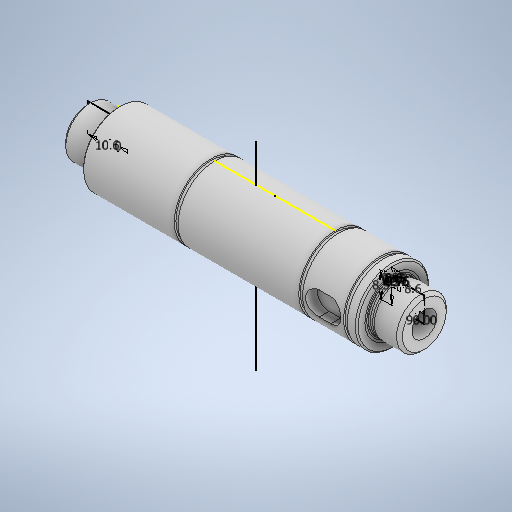
# Autodesk Inventor part: 26-10-204
Saved by Autodesk Inventor 2025.2 (Build 292293000, 293)
## iProperties
Created: 2024-12-02
Part Number: 26-10-204
Material: Generic
Document SubType Name: Modeling
Designer: Zvonko.Gabric
Density: 1 g/cm^3
Appearance: Default
Author: Zvonko.Gabric
Autodesk Inventor part; units mm, degrees
ref_plane "YZ Plane" through (0, 0, 0) normal (1, 0, 0) x (0, 1, 0)
ref_plane "XZ Plane" through (0, 0, 0) normal (0, 1, 0) x (-1, 0, 0)
sketch "Sketch1" plane through (0, 0, 0) normal (0, 1, 0) x (-1, 0, 0)
  line L0 (0, 0) -> (93.8, 0)
  line L1 (0, 9.695) -> (0.1, 8.9835)
  line L2 (0, 12.5) -> (0, 9.695)
  line L3 (3.2, 12.5) -> (0, 12.5)
  line L4 (3.2, 11.95) -> (3.2, 12.5)
  line L5 (4.5, 11.95) -> (3.2, 11.95)
  line L6 (4.5, 12.5) -> (4.5, 11.95)
  line L7 (18.5, 12.5) -> (4.5, 12.5)
  line L8 (18.5, 11.95) -> (18.5, 12.5)
  line L9 (19.8, 11.95) -> (18.5, 11.95)
  line L10 (19.8, 12.5) -> (19.8, 11.95)
  line L11 (61, 12.5) -> (19.8, 12.5)
  line L12 (61, 11.95) -> (61, 12.5)
  line L13 (62.3, 11.95) -> (61, 11.95)
  line L14 (62.3, 12.5) -> (62.3, 11.95)
  line L15 (93.8, 12.5) -> (62.3, 12.5)
  line L16 (93.8, 9.695) -> (93.8, 12.5)
  line L17 (93.7, 8.9835) -> (93.8, 9.695)
  line L18 (93.8, 0) -> (93.8, 8.5597)
  line L19 (0, 0) -> (93.8, 0)
  line L20 (0, 8.5597) -> (0, 0)
  arc A0 (0, 8.5597) -> (0.1, 8.9835) centre (-0.4942, 8.9) ccw
  arc A1 (93.7, 8.9835) -> (93.8, 8.5597) centre (94.2942, 8.9) ccw
  dimension "d0" = 0
  dimension "d1" = 12.5
  dimension "d2" = 8.5597
  dimension "d3" = 2.805
  dimension "d4" = 0.7185
  dimension "d5" = 0.6
  dimension "d6" = 3.2
  dimension "d7" = 0.55
  dimension "d8" = 1.3
  dimension "d9" = 0.55
  dimension "d10" = 14
  dimension "d11" = 0.55
  dimension "d12" = 1.3
  dimension "d13" = 0.55
  dimension "d14" = 41.2
  dimension "d15" = 0.55
  dimension "d16" = 1.3
  dimension "d17" = 0.55
  dimension "d18" = 31.5
  dimension "d19" = 2.805
  dimension "d20" = 0.7115
  dimension "d21" = 0.6
  dimension "d22" = 8.5597
  dimension "d23" = 93.8
  dimension "d24" = 90
  dimension "d25" = 90
  dimension "d26" = 90
  dimension "d27" = 90
  dimension "d28" = 90
  dimension "d29" = 90
  dimension "d30" = 90
  dimension "d31" = 90
  dimension "d32" = 90
  dimension "d33" = 90
  constraints: 42 end point, 4 point on circle, 2 centre point
  measures "d0" distance of point (0, 0) L0.start
  measures "d1" distance between parallel lines of L3 L0
  measures "d2" distance of L20.start L0.start
  measures "d3" distance of L2.start L1.start
  measures "d4" distance of L1.start L1.end
  measures "d5" radius of A0
  measures "d6" distance of L3.start L2.start
  measures "d7" distance of L4.start L3.start
  measures "d8" distance of L5.start L4.start
  measures "d9" distance of L6.start L5.start
  measures "d10" distance of L7.start L6.start
  measures "d11" distance of L8.start L7.start
  measures "d12" distance of L9.start L8.start
  measures "d13" distance of L10.start L9.start
  measures "d14" distance of L11.start L10.start
  measures "d15" distance of L12.start L11.start
  measures "d16" distance of L13.start L12.start
  measures "d17" distance of L14.start L13.start
  measures "d18" distance of L15.start L14.start
  measures "d19" distance of L16.start L15.start
  measures "d20" vertical distance of L17.start L16.start
  measures "d21" radius of A1
  measures "d22" distance of L0.end L18.end
  measures "d23" distance of L0.start L0.end
  measures "d24" angle of L2 L3
  measures "d25" angle of L0 L20
  measures "d26" angle of L3 L4
  measures "d27" angle of L7 L6
  measures "d28" angle of L7 L8
  measures "d29" angle of L11 L10
  measures "d30" angle of L12 L11
  measures "d31" angle of L15 L14
  measures "d32" angle of L15 L16
  measures "d33" angle of L0 L18
revolve "Revolution1" add sketch "Sketch1" angle 360 about axis through (0, 0, 0) along (-1, 0, 0)
sketch "Sketch2" plane through (0, 0, 0) normal (0, 0, 1) x (1, 0, 0)
  line L0 (0, 0) -> (-0.1, 8.4994)
  line L1 (0, 0) -> (-0.01, 8.5)
  line L2 (-0.01, 8.5) -> (0.04, 8.5)
  line L3 (0.04, 8.5) -> (0.04, 8.3) construction
  line L4 (0.04, 8.3) -> (0.49, 8.3) construction
  arc A0 (0.04, 8.5) -> (0.49, 8.3) centre (0.4872, 8.9) ccw
  line L5 (0.49, 8.3) -> (1.25, 8.3)
  line L6 (1.25, 8.3) -> (2, 8.3) construction
  line L7 (2, 8.3) -> (2, 8.5) construction
  line L8 (2, 8.5) -> (10.6, 8.5)
  line L9 (10.6, 8.5) -> (10.6, 0)
  line L10 (10.6, 0) -> (0, 0)
  line L11 (-19.8, 12.5) -> (-61, 12.5) projected
  line L12 (-40.4, 12.5) -> (-40.4, -12.5)
  line L13 (-19.8, -12.5) -> (-61, -12.5) projected
  line L14 (-46.9, 25.3625) -> (-46.9, -42.5251)
  line L15 (-93.8, 12.5) -> (-93.8, -12.5) projected
  line L16 (2, 8.5) -> (1.25, 8.3)
  line L17 (-93.8, 0) -> (-93.79, 8.5)
  line L18 (-93.79, 8.5) -> (-93.84, 8.5)
  line L19 (-93.84, 8.5) -> (-93.84, 8.3) construction
  line L20 (-93.84, 8.3) -> (-94.29, 8.3) construction
  arc A1 (-94.29, 8.3) -> (-93.84, 8.5) centre (-94.2872, 8.9) ccw
  line L21 (-94.29, 8.3) -> (-95.05, 8.3)
  line L22 (-95.05, 8.3) -> (-95.8, 8.3) construction
  line L23 (-95.8, 8.3) -> (-95.8, 8.5) construction
  line L24 (-95.8, 8.5) -> (-104.4, 8.5)
  line L25 (-104.4, 8.5) -> (-104.4, 0)
  line L26 (-104.4, 0) -> (-93.8, 0)
  line L27 (-95.8, 8.5) -> (-95.05, 8.3)
  dimension "d35" = 8.5
  dimension "d36" = 8.5
  dimension "d37" = 0.05
  dimension "d38" = 0.2
  dimension "d39" = 0.45
  dimension "d40" = 0.6
  dimension "d41" = 0.76
  dimension "d42" = 0.75
  dimension "d43" = 0.2
  dimension "d44" = 8.6
  dimension "d45" = 90
  dimension "d60" = 10.6
  dimension "d61" = 0
  constraints: 50 end point, 11 symmetric about line, 5 horizontal, 4 point on circle, 2 centre point, 2 midpoint, 2 perpendicular, 2 vertical, 1 other
  measures "d35" distance of L0.start L0.end
  measures "d36" distance of L0.start L1.end
  measures "d37" distance of L1.end L2.end
  measures "d38" distance of L2.end L3.end
  measures "d39" distance of L3.end L4.end
  measures "d40" radius of A0
  measures "d41" distance of L4.end L5.end
  measures "d42" distance of L5.end L6.end
  measures "d43" distance of L6.end L7.end
  measures "d44" distance of L7.end L8.end
  measures "d45" angle of L10 L9
  measures "d60" distance of L26.start L26.end
  measures "d61" distance from line of L26.end L15
revolve "Revolution2" add sketch "Sketch2" angle 360 about axis through (10.6, 0, 0) along (-1, 0, 0) contours L1 L2 A0 L5 L16 L8 L9 L10 | L18 L17 L15 | L15 L26 L25 L24 L27 L21 A1 L18
chamfer "Chamfer1" distance 1 angle 45 1 edges at (10.6, -8.5, 0) measured on face at (4.8667, 8.4724, 0.684)
chamfer "Chamfer2" distance 1 angle 45 1 edges at (-104.4, -8.5, 0) measured on face at (-98.6667, 8.4724, 0.684)
chamfer "Chamfer3" distance 0.5 angle 45 1 edges at (0, 0, -12.5) measured on face at (-2.1333, -2.0051, 12.3381)
chamfer "Chamfer4" distance 0.5 angle 45 1 edges at (-93.8, 0, -12.5) measured on face at (-83.3, -1.0058, 12.4595)
sketch "Sketch3" plane through (0, 0, 0) normal (0, 0, 1) x (1, 0, 0)
  point P0 (0, 0)
ref_plane "Work Plane1" through (0, 0, 12.5) normal (0, 0, 1) x (1, 0, 0)
sketch "Sketch4" plane through (0, 0, 12.5) normal (0, 0, 1) x (1, 0, 0)
  line L0 (-13.5, 0) -> (-9.5, 0) construction
  line L1 (-13.5, 4) -> (-9.5, 4)
  line L2 (-9.5, -4) -> (-13.5, -4)
  arc A0 (-13.5, 4) -> (-13.5, -4) centre (-13.5, 0) ccw
  arc A1 (-9.5, -4) -> (-9.5, 4) centre (-9.5, 0) ccw
  line L3 (10.6, 7.5) -> (10.6, -7.5) projected
  point P0 (0, 0)
  point P1 (-11.5, 0)
  point P2 (-5.5, 0)
  point P3 (-17.5, 0)
  dimension "d63" = 12
  dimension "d64" = 8
  dimension "d65" = 16.1
  dimension "d66" = 0
  constraints: 8 end point, 6 point on circle, 4 tangent, 2 centre point, 1 horizontal, 1 midpoint, 1 parallel
  measures "d63" distance of point (-5.5, 0) point (-17.5, 0)
  measures "d64" distance between parallel lines of L2 L1
  measures "d65" distance from line of L3 point (-5.5, 0)
  measures "d66" vertical distance of point (0, 0) point (-11.5, 0)
extrude "Extrusion1" cut sketch "Sketch4" against normal blind 4
sketch "Sketch5" plane through (10.6, 0, 0) normal (1, 0, 0) x (0, 0, -1)
  point P0 (0, 0)
hole "Hole1" at (10.6, 0, 0) direction (-1, 0, 0) diameter 4 depth 6.47 tip angle 118 countersink diameter 8.5 countersink angle 60
sketch "Sketch6" plane through (-104.4, 0, 0) normal (-1, 0, 0) x (0, 0, 1)
  point P0 (0, 0)
hole "Hole2" at (-104.4, 0, 0) direction (1, 0, 0) diameter 4 depth 6.47 tip angle 118 countersink diameter 8.5 countersink angle 60
body "Solid1"
